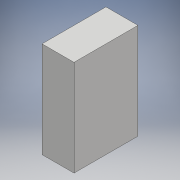
# Autodesk Inventor part: FlanecPodGayku
Saved by Autodesk Inventor 2017 (Build 210142000, 142)
## iProperties
Part Number: FlanecPodGayku
Material: Типовые
Document SubType Name: Modeling
Designer: Nikita
Density: 1 g/cm^3
Appearance: По умолчанию
Author: Nikita
## iProperties of the stored document FlanecPodGayku_3DПЕЧАТЬ.ipt
Part Number: FlanecPodGayku_3DПЕЧАТЬ
Material: Типовые
Document SubType Name: Modeling
Designer: Nikita
Density: 1 g/cm^3
Appearance: По умолчанию
Author: Nikita
Autodesk Inventor part; units mm, degrees
ref_plane "YZ Plane" through (0, 0, 0) normal (1, 0, 0) x (0, 1, 0)
ref_plane "XZ Plane" through (0, 0, 0) normal (0, 1, 0) x (-1, 0, 0)
ref_plane "XY Plane" through (0, 0, 0) normal (0, 0, 1) x (1, 0, 0)
sketch "Эскиз1" plane through (0, 0, 0) normal (0, 1, 0) x (-1, 0, 0)
  line L0 (0, 0) -> (10, 0)
  line L1 (10, 0) -> (10, -30)
  line L2 (10, -30) -> (0, -30)
  line L3 (0, -30) -> (0, 0)
  dimension "d0" = 10
  dimension "d1" = 30
  constraints: 8 end point, 2 parallel, 1 horizontal, 1 perpendicular
  measures "d0" distance of L1.end L2.end
  measures "d1" distance of L0.end L1.end
extrude "Выдавливание1" add sketch "Эскиз1" along normal blind 20
sketch "Эскиз2" plane through (0, 20, 0) normal (0, 1, 0) x (1, 0, 0)
  line L0 (-7.0207, 11.5) -> (-9.0415, 15)
  line L1 (-9.0415, 15) -> (-7.0207, 18.5)
  line L2 (-7.0207, 18.5) -> (-2.9793, 18.5)
  line L3 (-2.9793, 18.5) -> (-0.9585, 15)
  line L4 (-0.9585, 15) -> (-2.9793, 11.5)
  line L5 (-2.9793, 11.5) -> (-7.0207, 11.5)
  line L6 (-10, 30) -> (-10, 0) projected
  line L7 (0, 30) -> (-10, 30) projected
  point P0 (0, 0)
  point P1 (-5, 15)
  point P2 (-10, 15)
  point P3 (-5, 30)
  dimension "d4" = 3.5
  constraints: 12 end point, 2 horizontal alignment, 2 midpoint, 1 vertical alignment, 13 other
  measures "d4" distance from line of L5 point (-5, 15)
sketch "Эскиз3" plane through (0, 20, 0) normal (0, 1, 0) x (1, 0, 0)
  circle A0 centre (-5, 15) radius 2
  point P0 (0, 0)
  dimension "d5" = 4
  constraints: 1 centre point, 1 coincident
  measures "d5" diameter of A0
extrude "Выдавливание2" cut sketch "Эскиз3" against normal blind 10
extrude "Выдавливание3" cut sketch "Эскиз2" against normal blind 3.2
